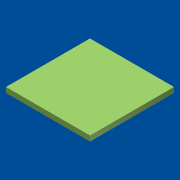
# Autodesk Inventor part: Tripod_Table
Saved by Autodesk Inventor 2014 (Build 180170000, 170)
## iProperties
Created: 2009-02-09
Part Number: Tripod_Table
Document SubType Name: Modeling
Designer: lminardi
Density: 0.899 g/cm^3
Material: Polypropylene
Appearance: Smooth - White
Author: lminardi
Autodesk Inventor part; units mm, degrees
ref_plane "YZ Plane" through (0, 0, 0) normal (1, 0, 0) x (0, 1, 0)
ref_plane "XZ Plane" through (0, 0, 0) normal (0, 1, 0) x (-1, 0, 0)
ref_plane "XY Plane" through (0, 0, 0) normal (0, 0, 1) x (1, 0, 0)
sketch "SketchTable" plane through (0, 0, 0) normal (0, 1, 0) x (-1, 0, 0)
  line L0 (0, 0) -> (-203.2, 0)
  line L1 (-203.2, 0) -> (-203.2, 203.2)
  line L2 (-203.2, 203.2) -> (0, 203.2)
  line L3 (0, 203.2) -> (0, 0)
  dimension "d0" = 203.2
  dimension "d1" = 203.2
  constraints: 8 end point, 2 parallel, 1 horizontal, 1 perpendicular, 1 other
  measures "d0" distance of L2.end L0.start
  measures "d1" distance of L0.start L0.end
extrude "Extrusion1" add sketch "SketchTable" along normal blind 12.7
body "Solid1"
